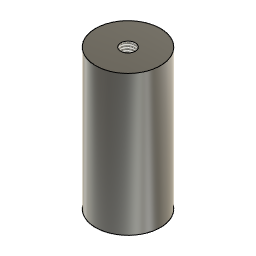
Spool Centre v2 (Autodesk Fusion 360 design; units mm, degrees)
Autodesk Fusion 360 part; units mm, degrees
sketch "Sketch1" plane through (0, 0, 0) normal (0, 0, 1) x (1, 0, 0)
  circle A0 centre (0, 0) radius 15
  dimension "d1" = 30
  constraint coincident A0.centre origin
  measures "d1" diameter of A0
extrude "Extrude1" add sketch "Sketch1" along normal blind 65
hole "Hole1" at (0, 0, 65) direction (0, 0, -1) diameter 6.78 depth 25 tip angle 180
thread "Thread1" "ISO Metric profile 8.0 M8x1.25 6H"
hole "Hole2" at (0, 0, 0) direction (0, 0, 1) diameter 6.78 depth 25 tip angle 180
thread "Thread2" "ISO Metric profile 8.0 M8x1.25 6H"
